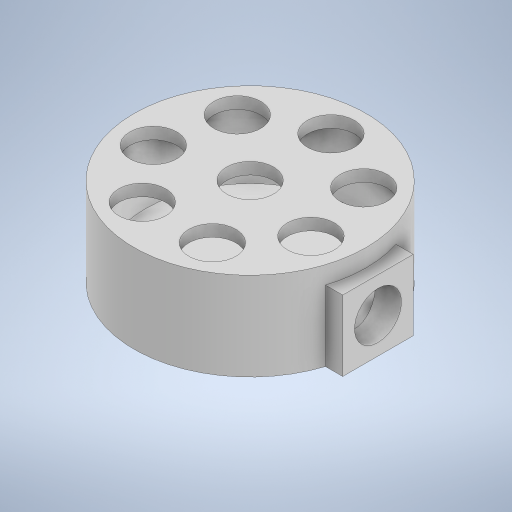
# Autodesk Inventor part: braided_input_connector_3.2mm_8ea
Saved by Autodesk Inventor 2024 (Build 280153000, 153)
## iProperties
Created: 2024-07-10
Part Number: braided_input_connector_3.2mm_8ea
Material: 일반
Document SubType Name: Modeling
Designer: Gihyeok Na
Density: 1 g/cm^3
Appearance: 기본값
Author: Gihyeok Na
Autodesk Inventor part; units mm, degrees
ref_plane "XZ Plane" through (0, 0, 0) normal (0, 1, 0) x (-1, 0, 0)
sketch "스케치1" plane through (0, 0, 0) normal (0, 1, 0) x (-1, 0, 0)
  circle A0 centre (0, 0) radius 5.5
  circle A1 centre (0, -5.5) radius 1.6
  circle A2 centre (4.3001, -3.4292) radius 1.6
  circle A3 centre (5.3621, 1.2239) radius 1.6
  circle A4 centre (2.3864, 4.9553) radius 1.6
  circle A5 centre (-2.3864, 4.9553) radius 1.6
  circle A6 centre (-5.3621, 1.2239) radius 1.6
  circle A7 centre (-4.3001, -3.4292) radius 1.6
  circle A8 centre (0, 0) radius 7.9
  circle A9 centre (0, 0) radius 1.6
  dimension "d0" = 11
  dimension "d1" = 3.2
  dimension "d4" = 360
  dimension "d6" = 15.8
  dimension "d7" = 3.2
  constraints: 9 centre point, 3 coincident, 1 vertical alignment, 17 other
  measures "d1" diameter of A1
  measures "d6" diameter of A8
  measures "d7" diameter of A9
extrude "돌출1" add sketch "스케치1" against normal blind 6 contours A0 A3 | A0 A3 | A3 A0 A2 A1 A7 A6 A5 A4 | A4 A0 | A0 A4 | A2 A0 | A0 A2 | A5 A0 | A0 A5 | A1 A0 | A0 A1 | A6 A0 | A0 A6 | A7 A0 | A0 A7 | A8 | A9
extrude "돌출2" cut sketch "스케치1" against normal blind 5.2 contours A0 A3 | A0 A3 | A4 A0 | A0 A4 | A2 A0 | A0 A2 | A5 A0 | A0 A5 | A1 A0 | A0 A1 | A6 A0 | A0 A6 | A7 A0 | A0 A7 | A9
ref_plane "작업 평면1" through (7.9, 0, 0) normal (1, 0, 0) x (0, 1, 0)
sketch "스케치2" plane through (7.9, 0, 0) normal (1, 0, 0) x (0, 1, 0)
  line L0 (-6, 7.9) -> (-6, -7.9) projected
  line L1 (0, -7.9) -> (0, 7.9) projected
  line L2 (-1.2, 2.4) -> (-6, 2.4)
  line L3 (-6, 2.4) -> (-6, -2.4)
  line L4 (-6, -2.4) -> (-1.2, -2.4)
  line L5 (-1.2, -2.4) -> (-1.2, 2.4)
  line L6 (-1.2, 2.4) -> (-6, -2.4) construction
  line L7 (-6, 2.4) -> (-1.2, -2.4) construction
  line L8 (0, 0) -> (-6, 0) construction
  circle A0 centre (-3.6, 0) radius 1.6
  point P0 (-6, -2.4)
  dimension "d12" = 4.8
  dimension "d13" = 4.8
  dimension "d14" = 3.2
  constraints: 14 end point, 3 midpoint, 2 parallel, 2 perpendicular, 1 centre point, 1 coincident, 1 collinear, 1 horizontal, 1 point on line
  measures "d12" distance of L4.end L3.end
  measures "d13" distance of L4.end L2.start
  measures "d14" diameter of A0
extrude "돌출3" add sketch "스케치2" against normal blind 0.6
ref_plane "작업 평면3" through (0, -5.2, 0) normal (0, -1, 0) x (1, 0, 0)
sketch "스케치5" plane through (0, -5.2, 0) normal (0, -1, 0) x (1, 0, 0)
  circle A0 centre (-5.3621, 1.2239) radius 1.6 projected
  circle A1 centre (4.3001, -3.4292) radius 1.6 projected
  circle A2 centre (-2.3864, 4.9553) radius 1.6 projected
  circle A3 centre (2.3864, 4.9553) radius 1.6 projected
  circle A4 centre (0, -5.5) radius 1.6 projected
  circle A5 centre (5.3621, 1.2239) radius 1.6 projected
  circle A6 centre (-5.3621, 1.2239) radius 1.6 projected
  circle A7 centre (0, 0) radius 1.6 projected
  circle A8 centre (-4.3001, -3.4292) radius 1.6 projected
  circle A9 centre (0, 0) radius 7.9 projected
  circle A10 centre (0, 0) radius 7.1
  constraints: 1 centre point, 1 coincident, 1 tangent
extrude "돌출4" cut sketch "스케치5" against normal blind 4.4 contours A0 | A8 | A4 | A1 | A5 | A3 | A2 | A10 | A7
extrude "돌출5" cut sketch "스케치2" against normal blind 1.85 contours A0
extrude "돌출6" add sketch "스케치2" along normal blind 0.8
sketch "스케치7" plane through (0, -6, 0) normal (0, -1, 0) x (1, 0, 0)
  circle A0 centre (0, 0) radius 2.7
  circle A1 centre (0, 0) radius 1.7
  dimension "d29" = 5.4
  dimension "d30" = 3.4
  constraints: 2 centre point, 2 coincident
  measures "d29" diameter of A0
  measures "d30" diameter of A1
extrude "돌출7" add sketch "스케치7" along normal blind 2.5
